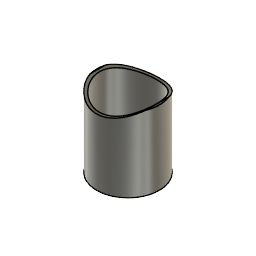
Support_Pipe (Autodesk Fusion 360 design; units mm, degrees)
part number: 2026-02-17-01-41-00-616
Autodesk Fusion 360 part; units mm, degrees
cylinder "CylinderPrimitive2" add diameter 40 height 50 placed x (1, 0, 0) y (0, 1, 0) z (0, 0, 1) at (84.4063, -23.6225, 0)
shell "Shell1" thickness 2 outward yes removed faces 1 at (89.1487, -30.7337, 50)
delete_face "DeleteFace1" 1 faces at (89.1487, -30.7337, 0)
sketch "Sketch3" plane through (0, 15, 0) normal (0, 1, 0) x (-1, 0, 0)
  circle A0 centre (-84, 87) radius 42.5
  circle A1 centre (-84, 87) radius 42.5
  constraint concentric A0 A1
extrude "Extrude1" cut sketch "Sketch3" against normal blind 80
